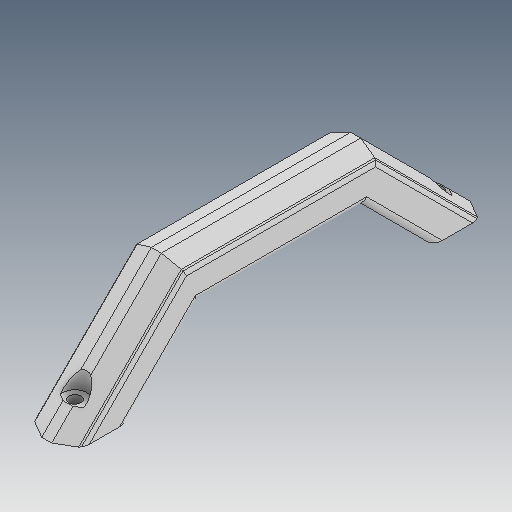
# Autodesk Inventor part: Handle
Saved by Autodesk Inventor 2027 (Build 310192060, 192F)
## iProperties
Created: 2026-07-28
Part Number: Handle
Material: Generic
Document SubType Name: Modeling
Designer: prest
Density: 1 g/cm^3
Appearance: Default
Author: prest
Autodesk Inventor part; units mm, degrees
ref_plane "YZ Plane" through (0, 0, 0) normal (1, 0, 0) x (0, 1, 0)
ref_plane "XY Plane" through (0, 0, 0) normal (0, 0, 1) x (1, 0, 0)
sketch "Sketch1" plane through (0, 0, 0) normal (1, 0, 0) x (0, 1, 0)
  line L0 (0, 105) -> (55, 50)
  line L1 (55, 50) -> (55, -50)
  line L2 (55, -50) -> (0, -105)
  line L3 (0, 105) -> (0, -115) construction
  line L4 (0, -76.7157) -> (35, -41.7157)
  line L5 (35, -41.7157) -> (35, 41.7157)
  line L6 (35, 41.7157) -> (0, 76.7157)
  line L7 (0, -115) -> (0, -76.7157)
  line L8 (0, 76.7157) -> (0, 105)
  point P0 (0, 0)
  point P1 (55, 0)
  point P2 (0, -5)
  point P3 (35, 0)
  point P4 (0, -105)
  dimension "d0" = 210
  dimension "d2" = 45
  dimension "d3" = 20
  dimension "d4" = 35
  dimension "d5" = 20
  constraints: 18 end point, 3 midpoint, 2 collinear, 2 horizontal alignment, 2 perpendicular, 2 point on line, 2 vertical, 2 vertical alignment
  measures "d0" distance of L2.end L0.start
  measures "d2" angle of L3 L0
  measures "d3" distance between parallel lines of L0 L6
  measures "d4" distance from line of point (0, -5) L5
  measures "d5" distance between parallel lines of L1 L5
extrude "Extrusion1" add sketch "Sketch1" along normal mid plane 25
chamfer "Chamfer1" distance 5 angle 45 6 edges at (-12.5, 27.5, -77.5) (-12.5, 55, 0) (-12.5, 27.5, 77.5) (12.5, 27.5, 77.5) (12.5, 55, 0) (12.5, 27.5, -77.5)
chamfer "Chamfer2" distance 5 angle 45 6 edges at (7.5, 27.5, 77.5) (-7.5, 27.5, 77.5) (-7.5, 55, 0) (7.5, 55, 0) (7.5, 27.5, -77.5) (-7.5, 27.5, -77.5)
fillet "Fillet1" radius 3 6 edges at (12.5, 25, 72.9289) (12.5, 50, 0) (12.5, 25, -72.9289) (-12.5, 25, -72.9289) (-12.5, 50, 0) (-12.5, 25, 72.9289)
fillet "Fillet2" radius 3 6 edges at (-12.5, 17.5, -59.2157) (-12.5, 35, 0) (-12.5, 17.5, 59.2157) (12.5, 17.5, 59.2157) (12.5, 35, 0) (12.5, 17.5, -59.2157)
sketch "Sketch2" plane through (-2.5, 0, 105) normal (0, -1, 0) x (1, 0, 0)
  line L0 (-7, -181.7157) -> (12, -181.7157) projected
  line L1 (0, -210) -> (5, -210) projected
  point P0 (2.5, -105)
  point P1 (2.5, -195.8579)
  point P2 (2.5, -181.7157)
  point P3 (2.5, -181.7157)
  point P4 (2.5, -210)
  dimension "d20" = 14.1421
  dimension "d22" = 28.2843
  constraints: 3 midpoint, 1 vertical alignment
  measures "d20" distance of point (2.5, -181.716) point (2.5, -195.858)
  measures "d22" distance of point (2.5, -181.716) point (2.5, -210)
hole "Hole1" at (0, 0, -90.8579) direction (0, 1, 0) diameter 6 end through all
ref_plane "Work Plane3" through (0, 17.1421, -87.8579) normal (0, 1, 0) x (-1, 0, 0)
sketch "Sketch6" plane through (0, 17.1421, -87.8579) normal (0, 1, 0) x (-1, 0, 0)
  arc A0 (-2.5, -4.6583) -> (2.5, -4.6583) centre (0, -3) ccw projected
  circle A1 centre (0, -3) radius 6
  point P0 (0, 87.8579)
  dimension "d37" = 12
  constraints: 1 centre point, 1 coincident
  measures "d37" diameter of A1
extrude "Extrusion4" cut sketch "Sketch6" along normal blind 3 and the other way blind 6.5
mirror "Mirror2" about plane through (0, 0, 0) normal (0, 0, 1) of "Extrusion4", "Hole1"
equation "\"d20\" = 0.5 * d22"
body "Solid1"
